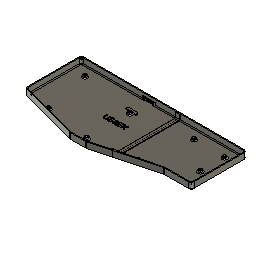
US8EK (Autodesk Fusion 360 design; units mm, degrees)
part number: 2026-03-01-18-28-36-830
Autodesk Fusion 360 part; units mm, degrees
(part 1 of 2)
sketch "Switch plate - imported" plane through (0, 0, 0) normal (0, 0, 1) x (1, 0, 0)
  line L0 (320.63607, 108.23641) -> (-5.90393, 108.23641)
  line L1 (-11.90393, 102.23641) -> (-11.90393, -1.458095)
  line L2 (-7.45498, -7.254149) -> (111.911453, -39.197144)
  line L3 (113.462504, -39.40109) -> (144.22489, -39.40109)
  line L4 (145.76596, -39.199805) -> (270.63368, -6.014874)
  line L5 (272.174751, -5.81359) -> (320.63607, -5.81359)
  line L6 (326.63607, 0.18641) -> (326.63607, 102.23641)
  arc A0 (-5.90393, 108.23641) -> (-11.90393, 102.23641) centre (-5.90393, 102.23641) ccw
  arc A1 (-11.90393, -1.458095) -> (-7.45498, -7.254149) centre (-5.90393, -1.458095) ccw
  arc A2 (111.911453, -39.197144) -> (113.462504, -39.40109) centre (113.462504, -33.40109) ccw
  arc A3 (144.22489, -39.40109) -> (145.76596, -39.199806) centre (144.22489, -33.40109) ccw
  arc A4 (272.174751, -5.81359) -> (270.63368, -6.014874) centre (272.174751, -11.81359) ccw
  arc A5 (320.63607, -5.81359) -> (326.63607, 0.18641) centre (320.63607, 0.18641) ccw
  arc A6 (326.63607, 102.23641) -> (320.63607, 108.23641) centre (320.63607, 102.23641) ccw
  line L7 (-8.820515, -4.494277) -> (4.494277, -8.820515)
  line L8 (4.494277, -8.820515) -> (8.820515, 4.494277)
  line L9 (8.820515, 4.494277) -> (-4.494277, 8.820515)
  line L10 (-4.494277, 8.820515) -> (-8.820515, -4.494277)
  line L11 (-2.949192, 13.575797) -> (10.3656, 9.249559)
  line L12 (10.3656, 9.249559) -> (14.691838, 22.56435)
  line L13 (14.691838, 22.56435) -> (1.377046, 26.890588)
  line L14 (1.377046, 26.890588) -> (-2.949192, 13.575797)
  line L15 (2.922131, 31.645871) -> (16.236923, 27.319633)
  line L16 (16.236923, 27.319633) -> (20.56316, 40.634424)
  line L17 (20.56316, 40.634424) -> (7.248369, 44.960662)
  line L18 (7.248369, 44.960662) -> (2.922131, 31.645871)
  line L19 (8.793454, 49.715945) -> (22.108245, 45.389707)
  line L20 (22.108245, 45.389707) -> (26.434483, 58.704498)
  line L21 (26.434483, 58.704498) -> (13.119692, 63.030736)
  line L22 (13.119692, 63.030736) -> (8.793454, 49.715945)
  line L23 (14.664777, 67.786019) -> (27.979568, 63.459781)
  line L24 (27.979568, 63.459781) -> (32.305806, 76.774572)
  line L25 (32.305806, 76.774572) -> (18.991015, 81.10081)
  line L26 (18.991015, 81.10081) -> (14.664777, 67.786019)
  line L27 (10.426914, -6.742074) -> (23.741705, -11.068312)
  line L28 (23.741705, -11.068312) -> (28.067943, 2.246479)
  line L29 (28.067943, 2.246479) -> (14.753152, 6.572717)
  line L30 (14.753152, 6.572717) -> (10.426914, -6.742074)
  line L31 (16.298237, 11.327999) -> (29.613028, 7.001762)
  line L32 (29.613028, 7.001762) -> (33.939266, 20.316553)
  line L33 (33.939266, 20.316553) -> (20.624475, 24.642791)
  line L34 (20.624475, 24.642791) -> (16.298237, 11.328)
  line L35 (22.16956, 29.398073) -> (35.484351, 25.071836)
  line L36 (35.484351, 25.071836) -> (39.810589, 38.386627)
  line L37 (39.810589, 38.386627) -> (26.495798, 42.712865)
  line L38 (26.495798, 42.712865) -> (22.16956, 29.398073)
  line L39 (28.040883, 47.468147) -> (41.355674, 43.141909)
  line L40 (41.355674, 43.141909) -> (45.681912, 56.456701)
  line L41 (45.681912, 56.456701) -> (32.36712, 60.782939)
  line L42 (32.36712, 60.782939) -> (28.040883, 47.468147)
  line L43 (33.912205, 65.538221) -> (47.226997, 61.211983)
  line L44 (47.226997, 61.211983) -> (51.553235, 74.526774)
  line L45 (51.553235, 74.526774) -> (38.238443, 78.853012)
  line L46 (38.238443, 78.853012) -> (33.912205, 65.538221)
  line L47 (32.617729, 0.068942) -> (45.932521, -4.257296)
  line L48 (45.932521, -4.257296) -> (50.258759, 9.057495)
  line L49 (50.258759, 9.057495) -> (36.943967, 13.383733)
  line L50 (36.943967, 13.383733) -> (32.617729, 0.068941)
  line L51 (38.489052, 18.139015) -> (51.803844, 13.812777)
  line L52 (51.803844, 13.812777) -> (56.130082, 27.127569)
  line L53 (56.130081, 27.127569) -> (42.81529, 31.453807)
  line L54 (42.81529, 31.453807) -> (38.489052, 18.139015)
  line L55 (44.360375, 36.209089) -> (57.675167, 31.882851)
  line L56 (57.675167, 31.882851) -> (62.001404, 45.197643)
  line L57 (62.001404, 45.197643) -> (48.686613, 49.52388)
  line L58 (48.686613, 49.52388) -> (44.360375, 36.209089)
  line L59 (50.231698, 54.279163) -> (63.546489, 49.952925)
  line L60 (63.546489, 49.952925) -> (67.872727, 63.267716)
  line L61 (67.872727, 63.267716) -> (54.557936, 67.593954)
  line L62 (54.557936, 67.593954) -> (50.231698, 54.279163)
  line L63 (56.103021, 72.349237) -> (69.417812, 68.022999)
  line L64 (69.417812, 68.022999) -> (73.74405, 81.33779)
  line L65 (73.74405, 81.33779) -> (60.429259, 85.664028)
  line L66 (60.429259, 85.664028) -> (56.103021, 72.349237)
  line L67 (53.042513, 1.444669) -> (66.357304, -2.881569)
  line L68 (66.357304, -2.881569) -> (70.683542, 10.433223)
  line L69 (70.683542, 10.433223) -> (57.368751, 14.759461)
  line L70 (57.368751, 14.759461) -> (53.042513, 1.444669)
  line L71 (58.913836, 19.514743) -> (72.228627, 15.188505)
  line L72 (72.228627, 15.188505) -> (76.554865, 28.503297)
  line L73 (76.554865, 28.503297) -> (63.240074, 32.829534)
  line L74 (63.240074, 32.829534) -> (58.913836, 19.514743)
  line L75 (64.785158, 37.584817) -> (78.09995, 33.258579)
  line L76 (78.09995, 33.258579) -> (82.426188, 46.57337)
  line L77 (82.426188, 46.57337) -> (69.111396, 50.899608)
  line L78 (69.111396, 50.899608) -> (64.785158, 37.584817)
  line L79 (70.656481, 55.654891) -> (83.971273, 51.328653)
  line L80 (83.971273, 51.328653) -> (88.297511, 64.643444)
  line L81 (88.297511, 64.643444) -> (74.982719, 68.969682)
  line L82 (74.982719, 68.969682) -> (70.656481, 55.654891)
  line L83 (76.527804, 73.724964) -> (89.842596, 69.398727)
  line L84 (89.842596, 69.398727) -> (94.168833, 82.713518)
  line L85 (94.168833, 82.713518) -> (80.854042, 87.039756)
  line L86 (80.854042, 87.039756) -> (76.527804, 73.724964)
  line L87 (68.757877, -11.673704) -> (82.072668, -15.999942)
  line L88 (82.072668, -15.999942) -> (86.398906, -2.685151)
  line L89 (86.398906, -2.685151) -> (73.084115, 1.641087)
  line L90 (73.084115, 1.641087) -> (68.757877, -11.673704)
  line L91 (74.6292, 6.396369) -> (87.943991, 2.070132)
  line L92 (87.943991, 2.070132) -> (92.270229, 15.384923)
  line L93 (92.270229, 15.384923) -> (78.955438, 19.711161)
  line L94 (78.955438, 19.711161) -> (74.6292, 6.396369)
  line L95 (80.500523, 24.466443) -> (93.815314, 20.140205)
  line L96 (93.815314, 20.140205) -> (98.141552, 33.454997)
  line L97 (98.141552, 33.454997) -> (84.826761, 37.781235)
  line L98 (84.826761, 37.781235) -> (80.500523, 24.466443)
  line L99 (86.371846, 42.536517) -> (99.686637, 38.210279)
  line L100 (99.686637, 38.210279) -> (104.012875, 51.52507)
  line L101 (104.012875, 51.525071) -> (90.698084, 55.851308)
  line L102 (90.698084, 55.851308) -> (86.371846, 42.536517)
  line L103 (92.243169, 60.606591) -> (105.55796, 56.280353)
  line L104 (105.55796, 56.280353) -> (109.884198, 69.595144)
  line L105 (109.884198, 69.595144) -> (96.569407, 73.921382)
  line L106 (96.569407, 73.921382) -> (92.243169, 60.606591)
  line L107 (85.650596, -21.168553) -> (98.965387, -25.49479)
  line L108 (98.965387, -25.49479) -> (103.291625, -12.179999)
  line L109 (103.291625, -12.179999) -> (89.976834, -7.853761)
  line L110 (89.976834, -7.853761) -> (85.650596, -21.168553)
  line L111 (91.521919, -3.098479) -> (104.83671, -7.424717)
  line L112 (104.83671, -7.424717) -> (109.162948, 5.890075)
  line L113 (109.162948, 5.890075) -> (95.848157, 10.216313)
  line L114 (95.848157, 10.216313) -> (91.521919, -3.098479)
  line L115 (97.393242, 14.971595) -> (110.708033, 10.645357)
  line L116 (110.708033, 10.645357) -> (115.034271, 23.960148)
  line L117 (115.034271, 23.960148) -> (101.71948, 28.286386)
  line L118 (101.71948, 28.286386) -> (97.393242, 14.971595)
  line L119 (103.264565, 33.041669) -> (116.579356, 28.715431)
  line L120 (116.579356, 28.715431) -> (120.905594, 42.030222)
  line L121 (120.905594, 42.030222) -> (107.590803, 46.35646)
  line L122 (107.590803, 46.35646) -> (103.264565, 33.041669)
  line L123 (109.135888, 51.111743) -> (122.450679, 46.785505)
  line L124 (122.450679, 46.785505) -> (126.776917, 60.100296)
  line L125 (126.776917, 60.100296) -> (113.462125, 64.426534)
  line L126 (113.462125, 64.426534) -> (109.135888, 51.111743)
  line L127 (103.94876, -27.455373) -> (113.316588, -37.8594)
  line L128 (113.316588, -37.8594) -> (123.720616, -28.491572)
  line L129 (123.720616, -28.491572) -> (114.352787, -18.087544)
  line L130 (114.352787, -18.087544) -> (103.94876, -27.455373)
  line L131 (109.050868, -10.797015) -> (122.365659, -15.123253)
  line L132 (122.365659, -15.123253) -> (126.691897, -1.808462)
  line L133 (126.691897, -1.808462) -> (113.377106, 2.517776)
  line L134 (113.377106, 2.517776) -> (109.050868, -10.797015)
  line L135 (-9.37893, 91.71141) -> (4.62107, 91.71141)
  line L136 (4.62107, 91.71141) -> (4.62107, 105.71141)
  line L137 (4.62107, 105.71141) -> (-9.37893, 105.71141)
  line L138 (-9.37893, 105.71141) -> (-9.37893, 91.71141)
  line L139 (13.48107, 91.71141) -> (27.48107, 91.71141)
  line L140 (27.48107, 91.71141) -> (27.48107, 105.71141)
  line L141 (27.48107, 105.71141) -> (13.48107, 105.71141)
  line L142 (13.48107, 105.71141) -> (13.48107, 91.71141)
  line L143 (32.48107, 91.71141) -> (46.48107, 91.71141)
  line L144 (46.48107, 91.71141) -> (46.48107, 105.71141)
  line L145 (46.48107, 105.71141) -> (32.48107, 105.71141)
  line L146 (32.48107, 105.71141) -> (32.48107, 91.71141)
  line L147 (51.48107, 91.71141) -> (65.48107, 91.71141)
  line L148 (65.48107, 91.71141) -> (65.48107, 105.71141)
  line L149 (65.48107, 105.71141) -> (51.48107, 105.71141)
  line L150 (51.48107, 105.71141) -> (51.48107, 91.71141)
  line L151 (70.48107, 91.71141) -> (84.48107, 91.71141)
  line L152 (84.48107, 91.71141) -> (84.48107, 105.71141)
  line L153 (84.48107, 105.71141) -> (70.48107, 105.71141)
  line L154 (70.48107, 105.71141) -> (70.48107, 91.71141)
  line L155 (93.34107, 91.71141) -> (107.34107, 91.71141)
  line L156 (107.34107, 91.71141) -> (107.34107, 105.71141)
  line L157 (107.34107, 105.71141) -> (93.34107, 105.71141)
  line L158 (93.34107, 105.71141) -> (93.34107, 91.71141)
  line L159 (112.34107, 91.71141) -> (126.34107, 91.71141)
  line L160 (126.34107, 91.71141) -> (126.34107, 105.71141)
  line L161 (126.34107, 105.71141) -> (112.34107, 105.71141)
  line L162 (112.34107, 105.71141) -> (112.34107, 91.71141)
  line L163 (131.34107, 91.71141) -> (145.34107, 91.71141)
  line L164 (145.34107, 91.71141) -> (145.34107, 105.71141)
  line L165 (145.34107, 105.71141) -> (131.34107, 105.71141)
  line L166 (131.34107, 105.71141) -> (131.34107, 91.71141)
  line L167 (150.34107, 91.71141) -> (164.34107, 91.71141)
  line L168 (164.34107, 91.71141) -> (164.34107, 105.71141)
  line L169 (164.34107, 105.71141) -> (150.34107, 105.71141)
  line L170 (150.34107, 105.71141) -> (150.34107, 91.71141)
  line L171 (173.20107, 91.71141) -> (187.20107, 91.71141)
  line L172 (187.20107, 91.71141) -> (187.20107, 105.71141)
  line L173 (187.20107, 105.71141) -> (173.20107, 105.71141)
  line L174 (173.20107, 105.71141) -> (173.20107, 91.71141)
  line L175 (192.20107, 91.71141) -> (206.20107, 91.71141)
  line L176 (206.20107, 91.71141) -> (206.20107, 105.71141)
  line L177 (206.20107, 105.71141) -> (192.20107, 105.71141)
  line L178 (192.20107, 105.71141) -> (192.20107, 91.71141)
  line L179 (211.20107, 91.71141) -> (225.20107, 91.71141)
  line L180 (225.20107, 91.71141) -> (225.20107, 105.71141)
  line L181 (225.20107, 105.71141) -> (211.20107, 105.71141)
  line L182 (211.20107, 105.71141) -> (211.20107, 91.71141)
  line L183 (230.20107, 91.71141) -> (244.20107, 91.71141)
  line L184 (244.20107, 91.71141) -> (244.20107, 105.71141)
  line L185 (244.20107, 105.71141) -> (230.20107, 105.71141)
  line L186 (230.20107, 105.71141) -> (230.20107, 91.71141)
  line L187 (272.11107, -3.28859) -> (286.11107, -3.28859)
  line L188 (286.11107, -3.28859) -> (286.11107, 10.71141)
  line L189 (286.11107, 10.71141) -> (272.11107, 10.71141)
  line L190 (272.11107, 10.71141) -> (272.11107, -3.28859)
  line L191 (272.11107, 15.71141) -> (286.11107, 15.71141)
  line L192 (286.11107, 15.71141) -> (286.11107, 29.71141)
  line L193 (286.11107, 29.71141) -> (272.11107, 29.71141)
  line L194 (272.11107, 29.71141) -> (272.11107, 15.71141)
  line L195 (281.63607, 34.71141) -> (295.63607, 34.71141)
  line L196 (295.63607, 34.71141) -> (295.63607, 48.71141)
  line L197 (295.63607, 48.71141) -> (281.63607, 48.71141)
  line L198 (281.63607, 48.71141) -> (281.63607, 34.71141)
  line L199 (272.11107, 53.71141) -> (286.11107, 53.71141)
  line L200 (286.11107, 53.71141) -> (286.11107, 67.71141)
  line L201 (286.11107, 67.71141) -> (272.11107, 67.71141)
  line L202 (272.11107, 67.71141) -> (272.11107, 53.71141)
  line L203 (281.63607, 72.71141) -> (295.63607, 72.71141)
  line L204 (295.63607, 72.71141) -> (295.63607, 86.71141)
  line L205 (295.63607, 86.71141) -> (281.63607, 86.71141)
  line L206 (281.63607, 86.71141) -> (281.63607, 72.71141)
  line L207 (272.11107, 91.71141) -> (286.11107, 91.71141)
  line L208 (286.11107, 91.71141) -> (286.11107, 105.71141)
  line L209 (286.11107, 105.71141) -> (272.11107, 105.71141)
  line L210 (272.11107, 105.71141) -> (272.11107, 91.71141)
  line L211 (291.11107, -3.28859) -> (305.11107, -3.28859)
  line L212 (305.11107, -3.28859) -> (305.11107, 10.71141)
  line L213 (305.11107, 10.71141) -> (291.11107, 10.71141)
  line L214 (291.11107, 10.71141) -> (291.11107, -3.28859)
  line L215 (291.11107, 15.71141) -> (305.11107, 15.71141)
  line L216 (305.11107, 15.71141) -> (305.11107, 29.71141)
  line L217 (305.11107, 29.71141) -> (291.11107, 29.71141)
  line L218 (291.11107, 29.71141) -> (291.11107, 15.71141)
  line L219 (291.11107, 53.71141) -> (305.11107, 53.71141)
  line L220 (305.11107, 53.71141) -> (305.11107, 67.71141)
  line L221 (305.11107, 67.71141) -> (291.11107, 67.71141)
  line L222 (291.11107, 67.71141) -> (291.11107, 53.71141)
  line L223 (291.11107, 91.71141) -> (305.11107, 91.71141)
  line L224 (305.11107, 91.71141) -> (305.11107, 105.71141)
  line L225 (305.11107, 105.71141) -> (291.11107, 105.71141)
  line L226 (291.11107, 105.71141) -> (291.11107, 91.71141)
  line L227 (310.11107, -3.28859) -> (324.11107, -3.28859)
  line L228 (324.11107, -3.28859) -> (324.11107, 10.71141)
  line L229 (324.11107, 10.71141) -> (310.11107, 10.71141)
  line L230 (310.11107, 10.71141) -> (310.11107, -3.28859)
  line L231 (310.11107, 15.71141) -> (324.11107, 15.71141)
  line L232 (324.11107, 15.71141) -> (324.11107, 29.71141)
  line L233 (324.11107, 29.71141) -> (310.11107, 29.71141)
  line L234 (310.11107, 29.71141) -> (310.11107, 15.71141)
  line L235 (310.11107, 34.71141) -> (324.11107, 34.71141)
  line L236 (324.11107, 34.71141) -> (324.11107, 48.71141)
  line L237 (324.11107, 48.71141) -> (310.11107, 48.71141)
  line L238 (310.11107, 48.71141) -> (310.11107, 34.71141)
  line L239 (310.11107, 53.71141) -> (324.11107, 53.71141)
  line L240 (324.11107, 53.71141) -> (324.11107, 67.71141)
  line L241 (324.11107, 67.71141) -> (310.11107, 67.71141)
  line L242 (310.11107, 67.71141) -> (310.11107, 53.71141)
  line L243 (310.11107, 72.71141) -> (324.11107, 72.71141)
  line L244 (324.11107, 72.71141) -> (324.11107, 86.71141)
  line L245 (324.11107, 86.71141) -> (310.11107, 86.71141)
  line L246 (310.11107, 86.71141) -> (310.11107, 72.71141)
  line L247 (310.11107, 91.71141) -> (324.11107, 91.71141)
  line L248 (324.11107, 91.71141) -> (324.11107, 105.71141)
  line L249 (324.11107, 105.71141) -> (310.11107, 105.71141)
  line L250 (310.11107, 105.71141) -> (310.11107, 91.71141)
  line L251 (-9.37893, 53.61141) -> (4.62107, 53.61141)
  line L252 (4.62107, 53.61141) -> (4.62107, 67.61141)
  line L253 (4.62107, 67.61141) -> (-9.37893, 67.61141)
  line L254 (-9.37893, 67.61141) -> (-9.37893, 53.61141)
  line L255 (-9.37893, 72.61141) -> (4.62107, 72.61141)
  line L256 (4.62107, 72.61141) -> (4.62107, 86.61141)
  line L257 (4.62107, 86.61141) -> (-9.37893, 86.61141)
  line L258 (-9.37893, 86.61141) -> (-9.37893, 72.61141)
  line L259 (255.305035, 48.586497) -> (268.619826, 52.912735)
  line L260 (268.619826, 52.912735) -> (264.293588, 66.227526)
  line L261 (264.293588, 66.227526) -> (250.978797, 61.901288)
  line L262 (250.978797, 61.901288) -> (255.305035, 48.586497)
  line L263 (249.433712, 66.656571) -> (262.748503, 70.982809)
  line L264 (262.748503, 70.982809) -> (258.422265, 84.2976)
  line L265 (258.422265, 84.2976) -> (245.107474, 79.971362)
  line L266 (245.107474, 79.971362) -> (249.433712, 66.656571)
  line L267 (253.06107, 91.71141) -> (267.06107, 91.71141)
  line L268 (267.06107, 91.71141) -> (267.06107, 105.71141)
  line L269 (267.06107, 105.71141) -> (253.06107, 105.71141)
  line L270 (253.06107, 105.71141) -> (253.06107, 91.71141)
  line L271 (121.86607, 7.89141) -> (135.86607, 7.89141)
  line L272 (135.86607, 7.89141) -> (135.86607, 21.89141)
  line L273 (135.86607, 21.89141) -> (121.86607, 21.89141)
  line L274 (121.86607, 21.89141) -> (121.86607, 7.89141)
  line L275 (112.34107, 72.66141) -> (126.34107, 72.66141)
  line L276 (126.34107, 72.66141) -> (126.34107, 86.66141)
  line L277 (126.34107, 86.66141) -> (112.34107, 86.66141)
  line L278 (112.34107, 86.66141) -> (112.34107, 72.66141)
  line L279 (131.34107, 72.66141) -> (145.34107, 72.66141)
  line L280 (145.34107, 72.66141) -> (145.34107, 86.66141)
  line L281 (145.34107, 86.66141) -> (131.34107, 86.66141)
  line L282 (131.34107, 86.66141) -> (131.34107, 72.66141)
  line L283 (253.933236, -8.820515) -> (267.248028, -4.494277)
  line L284 (267.248028, -4.494277) -> (262.92179, 8.820515)
  line L285 (262.92179, 8.820515) -> (249.606998, 4.494277)
  line L286 (249.606998, 4.494277) -> (253.933236, -8.820515)
  line L287 (248.061913, 9.249559) -> (261.376705, 13.575797)
  line L288 (261.376705, 13.575797) -> (257.050467, 26.890588)
  line L289 (257.050467, 26.890588) -> (243.735676, 22.56435)
  line L290 (243.735676, 22.56435) -> (248.061913, 9.249559)
  line L291 (242.19059, 27.319633) -> (255.505382, 31.645871)
  line L292 (255.505382, 31.645871) -> (251.179144, 44.960662)
  line L293 (251.179144, 44.960662) -> (237.864353, 40.634424)
  line L294 (237.864353, 40.634424) -> (242.19059, 27.319633)
  line L295 (236.319268, 45.389707) -> (249.634059, 49.715945)
  line L296 (249.634059, 49.715945) -> (245.307821, 63.030736)
  line L297 (245.307821, 63.030736) -> (231.99303, 58.704498)
  line L298 (231.99303, 58.704498) -> (236.319268, 45.389707)
  line L299 (230.447945, 63.459781) -> (243.762736, 67.786019)
  line L300 (243.762736, 67.786019) -> (239.436498, 81.10081)
  line L301 (239.436498, 81.10081) -> (226.121707, 76.774572)
  line L302 (226.121707, 76.774572) -> (230.447945, 63.459781)
  line L303 (234.685808, -11.068312) -> (248.000599, -6.742074)
  line L304 (248.000599, -6.742074) -> (243.674361, 6.572717)
  line L305 (243.674361, 6.572717) -> (230.35957, 2.246479)
  line L306 (230.35957, 2.246479) -> (234.685808, -11.068312)
  line L307 (228.814485, 7.001762) -> (242.129276, 11.327999)
  line L308 (242.129276, 11.327999) -> (237.803038, 24.642791)
  line L309 (237.803038, 24.642791) -> (224.488247, 20.316553)
  line L310 (224.488247, 20.316553) -> (228.814485, 7.001762)
  line L311 (222.943162, 25.071836) -> (236.257953, 29.398073)
  line L312 (236.257953, 29.398073) -> (231.931715, 42.712865)
  line L313 (231.931715, 42.712865) -> (218.616924, 38.386627)
  line L314 (218.616924, 38.386627) -> (222.943162, 25.071836)
  line L315 (217.071839, 43.141909) -> (230.38663, 47.468147)
  line L316 (230.38663, 47.468147) -> (226.060392, 60.782939)
  line L317 (226.060392, 60.782939) -> (212.745601, 56.456701)
  line L318 (212.745601, 56.456701) -> (217.071839, 43.141909)
  line L319 (211.200516, 61.211983) -> (224.515308, 65.538221)
  line L320 (224.515308, 65.538221) -> (220.18907, 78.853012)
  line L321 (220.18907, 78.853012) -> (206.874278, 74.526774)
  line L322 (206.874278, 74.526774) -> (211.200516, 61.211983)
  line L323 (212.494992, -4.257296) -> (225.809784, 0.068942)
  line L324 (225.809784, 0.068941) -> (221.483546, 13.383733)
  line L325 (221.483546, 13.383733) -> (208.168754, 9.057495)
  line L326 (208.168754, 9.057495) -> (212.494992, -4.257296)
  line L327 (206.623669, 13.812777) -> (219.938461, 18.139015)
  line L328 (219.938461, 18.139015) -> (215.612223, 31.453807)
  line L329 (215.612223, 31.453807) -> (202.297432, 27.127569)
  line L330 (202.297432, 27.127569) -> (206.623669, 13.812777)
  line L331 (200.752347, 31.882851) -> (214.067138, 36.209089)
  line L332 (214.067138, 36.209089) -> (209.7409, 49.52388)
  line L333 (209.7409, 49.52388) -> (196.426109, 45.197643)
  line L334 (196.426109, 45.197643) -> (200.752347, 31.882851)
  line L335 (194.881024, 49.952925) -> (208.195815, 54.279163)
  line L336 (208.195815, 54.279163) -> (203.869577, 67.593954)
  line L337 (203.869577, 67.593954) -> (190.554786, 63.267716)
  line L338 (190.554786, 63.267716) -> (194.881024, 49.952925)
  line L339 (189.009701, 68.022999) -> (202.324492, 72.349237)
  line L340 (202.324492, 72.349237) -> (197.998254, 85.664028)
  line L341 (197.998254, 85.664028) -> (184.683463, 81.33779)
  line L342 (184.683463, 81.33779) -> (189.009701, 68.022999)
  line L343 (192.070209, -2.881569) -> (205.385, 1.444669)
  line L344 (205.385, 1.444669) -> (201.058762, 14.759461)
  line L345 (201.058762, 14.759461) -> (187.743971, 10.433223)
  line L346 (187.743971, 10.433223) -> (192.070209, -2.881569)
  line L347 (186.198886, 15.188505) -> (199.513677, 19.514743)
  line L348 (199.513677, 19.514743) -> (195.187439, 32.829534)
  line L349 (195.18744, 32.829534) -> (181.872648, 28.503297)
  line L350 (181.872648, 28.503297) -> (186.198886, 15.188505)
  line L351 (180.327563, 33.258579) -> (193.642355, 37.584817)
  line L352 (193.642354, 37.584817) -> (189.316117, 50.899608)
  line L353 (189.316117, 50.899608) -> (176.001325, 46.57337)
  line L354 (176.001325, 46.57337) -> (180.327563, 33.258579)
  line L355 (174.45624, 51.328653) -> (187.771032, 55.654891)
  line L356 (187.771032, 55.654891) -> (183.444794, 68.969682)
  line L357 (183.444794, 68.969682) -> (170.130002, 64.643444)
  line L358 (170.130002, 64.643444) -> (174.45624, 51.328653)
  line L359 (168.584917, 69.398727) -> (181.899709, 73.724964)
  line L360 (181.899709, 73.724964) -> (177.573471, 87.039756)
  line L361 (177.573471, 87.039756) -> (164.258679, 82.713518)
  line L362 (164.258679, 82.713518) -> (168.584917, 69.398727)
  line L363 (176.354845, -15.999942) -> (189.669636, -11.673704)
  line L364 (189.669636, -11.673704) -> (185.343398, 1.641087)
  line L365 (185.343398, 1.641087) -> (172.028607, -2.685151)
  line L366 (172.028607, -2.685151) -> (176.354845, -15.999942)
  line L367 (170.483522, 2.070132) -> (183.798313, 6.39637)
  line L368 (183.798313, 6.396369) -> (179.472075, 19.711161)
  line L369 (179.472075, 19.711161) -> (166.157284, 15.384923)
  line L370 (166.157284, 15.384923) -> (170.483522, 2.070132)
  line L371 (164.612199, 20.140205) -> (177.92699, 24.466443)
  line L372 (177.92699, 24.466443) -> (173.600752, 37.781235)
  line L373 (173.600752, 37.781235) -> (160.285961, 33.454997)
  line L374 (160.285961, 33.454997) -> (164.612199, 20.140205)
  line L375 (158.740876, 38.210279) -> (172.055667, 42.536517)
  line L376 (172.055667, 42.536517) -> (167.729429, 55.851308)
  line L377 (167.729429, 55.851308) -> (154.414638, 51.525071)
  line L378 (154.414638, 51.525071) -> (158.740876, 38.210279)
  line L379 (152.869553, 56.280353) -> (166.184344, 60.606591)
  line L380 (166.184344, 60.606591) -> (161.858107, 73.921382)
  line L381 (161.858107, 73.921382) -> (148.543315, 69.595144)
  line L382 (148.543315, 69.595144) -> (152.869553, 56.280353)
  line L383 (159.462126, -25.49479) -> (172.776917, -21.168552)
  line L384 (172.776917, -21.168553) -> (168.450679, -7.853761)
  line L385 (168.450679, -7.853761) -> (155.135888, -12.179999)
  line L386 (155.135888, -12.179999) -> (159.462126, -25.49479)
  line L387 (153.590803, -7.424717) -> (166.905594, -3.098479)
  line L388 (166.905594, -3.098479) -> (162.579356, 10.216313)
  line L389 (162.579356, 10.216313) -> (149.264565, 5.890075)
  line L390 (149.264565, 5.890075) -> (153.590803, -7.424717)
  line L391 (147.71948, 10.645357) -> (161.034271, 14.971595)
  line L392 (161.034271, 14.971595) -> (156.708033, 28.286386)
  line L393 (156.708033, 28.286386) -> (143.393242, 23.960148)
  line L394 (143.393242, 23.960148) -> (147.71948, 10.645357)
  line L395 (141.848157, 28.715431) -> (155.162948, 33.041669)
  line L396 (155.162948, 33.041669) -> (150.83671, 46.35646)
  line L397 (150.83671, 46.35646) -> (137.521919, 42.030222)
  line L398 (137.521919, 42.030222) -> (141.848157, 28.715431)
  line L399 (135.976834, 46.785505) -> (149.291625, 51.111743)
  line L400 (149.291625, 51.111743) -> (144.965387, 64.426534)
  line L401 (144.965387, 64.426534) -> (131.650596, 60.100296)
  line L402 (131.650596, 60.100296) -> (135.976834, 46.785505)
  line L403 (145.110925, -37.8594) -> (154.478753, -27.455373)
  line L404 (154.478753, -27.455373) -> (144.074726, -18.087544)
  line L405 (144.074726, -18.087544) -> (134.706897, -28.491572)
  line L406 (134.706897, -28.491572) -> (145.110925, -37.8594)
  line L407 (136.061853, -15.123253) -> (149.376645, -10.797015)
  line L408 (149.376645, -10.797015) -> (145.050407, 2.517776)
  line L409 (145.050407, 2.517776) -> (131.735616, -1.808462)
  line L410 (131.735616, -1.808462) -> (136.061853, -15.123253)
  circle A7 centre (17.958543, 86.094258) radius 1.2
  circle A8 centre (37.317502, -8.11912) radius 1.2
  circle A9 centre (128.86607, -21.30359) radius 1.2
  circle A10 centre (128.86607, 66.32641) radius 1.2
  circle A11 centre (240.468971, 86.094258) radius 1.2
  circle A12 centre (221.110011, -8.11912) radius 1.2
  circle A13 centre (303.77607, 85.42641) radius 1.2
  circle A14 centre (303.77607, 35.99641) radius 1.2
  line L411 (-9.90393, 102.23641) -> (-9.90393, -1.458095)
  arc A15 (-9.90393, -1.458095) -> (-6.937964, -5.322131) centre (-5.90393, -1.458095) ccw
  line L412 (-6.937964, -5.322131) -> (112.42847, -37.265126)
  arc A16 (112.42847, -37.265126) -> (113.462504, -37.40109) centre (113.462504, -33.40109) ccw
  line L413 (113.462504, -37.40109) -> (144.22489, -37.40109)
  arc A17 (144.22489, -37.40109) -> (145.25227, -37.2669) centre (144.22489, -33.40109) ccw
  line L414 (145.25227, -37.2669) -> (270.11999, -4.081969)
  arc A18 (272.174751, -3.81359) -> (270.11999, -4.081969) centre (272.174751, -11.81359) ccw
  line L415 (272.174751, -3.81359) -> (320.63607, -3.81359)
  arc A19 (320.63607, -3.81359) -> (324.63607, 0.18641) centre (320.63607, 0.18641) ccw
  line L416 (324.63607, 0.18641) -> (324.63607, 102.23641)
  arc A20 (324.63607, 102.23641) -> (320.63607, 106.23641) centre (320.63607, 102.23641) ccw
  line L417 (320.63607, 106.23641) -> (-5.90393, 106.23641)
  arc A21 (-5.90393, 106.23641) -> (-9.90393, 102.23641) centre (-5.90393, 102.23641) ccw
  dimension "wall_thickness" = -2
sketch "Case - top down" plane through (0, 0, 0) normal (0, 0, 1) x (1, 0, 0)
  line L0 (-9.90393, 102.23641) -> (-9.90393, -1.458095)
  line L1 (-11.90393, 102.23641) -> (-11.90393, -1.458095)
  arc A0 (-11.90393, -1.458095) -> (-7.45498, -7.254149) centre (-5.90393, -1.458095) ccw
  arc A1 (-9.90393, -1.458095) -> (-6.937964, -5.322131) centre (-5.90393, -1.458095) ccw
  line L2 (-6.937964, -5.322131) -> (112.42847, -37.265126)
  line L3 (-7.45498, -7.254149) -> (111.911453, -39.197144)
  arc A2 (-5.90393, 106.23641) -> (-9.90393, 102.23641) centre (-5.90393, 102.23641) ccw
  arc A3 (-5.90393, 108.23641) -> (-11.90393, 102.23641) centre (-5.90393, 102.23641) ccw
  line L4 (320.63607, 106.23641) -> (-5.90393, 106.23641)
  line L5 (320.63607, 108.23641) -> (-5.90393, 108.23641)
  line L6 (113.462504, -37.40109) -> (144.22489, -37.40109)
  line L7 (113.462504, -39.40109) -> (144.22489, -39.40109)
  arc A4 (111.911453, -39.197144) -> (113.462504, -39.40109) centre (113.462504, -33.40109) ccw
  arc A5 (112.42847, -37.265126) -> (113.462504, -37.40109) centre (113.462504, -33.40109) ccw
  arc A6 (144.22489, -39.40109) -> (145.76596, -39.199806) centre (144.22489, -33.40109) ccw
  line L8 (145.76596, -39.199805) -> (270.63368, -6.014874)
  line L9 (145.25227, -37.2669) -> (270.11999, -4.081969)
  arc A7 (144.22489, -37.40109) -> (145.25227, -37.2669) centre (144.22489, -33.40109) ccw
  arc A8 (272.174751, -3.81359) -> (270.11999, -4.081969) centre (272.174751, -11.81359) ccw
  arc A9 (272.174751, -5.81359) -> (270.63368, -6.014874) centre (272.174751, -11.81359) ccw
  line L10 (272.174751, -5.81359) -> (320.63607, -5.81359)
  line L11 (272.174751, -3.81359) -> (320.63607, -3.81359)
  arc A10 (320.63607, -5.81359) -> (326.63607, 0.18641) centre (320.63607, 0.18641) ccw
  arc A11 (320.63607, -3.81359) -> (324.63607, 0.18641) centre (320.63607, 0.18641) ccw
  line L12 (324.63607, 0.18641) -> (324.63607, 102.23641)
  line L13 (326.63607, 0.18641) -> (326.63607, 102.23641)
  arc A12 (326.63607, 102.23641) -> (320.63607, 108.23641) centre (320.63607, 102.23641) ccw
  arc A13 (324.63607, 102.23641) -> (320.63607, 106.23641) centre (320.63607, 102.23641) ccw
sketch "Case - side" plane through (0, 0, 0) normal (1, 0, 0) x (0, 1, 0)
  line L0 (102.23641, 0) -> (-1.458095, 0) construction
  line L1 (-1.458095, 0) -> (-1.458095, 12)
  line L2 (-1.458095, 0) -> (-1.458095, -1.4)
  point P0 (-1.458095, 4)
  dimension "d2" = 12
  dimension "d3" = 1.4
  dimension "d28" = 4
  constraint perpendicular L0 L1
  constraint perpendicular L0 L2
extrude "Extrude1" add sketch "Case - top down" against normal up to surface (1.4 mm away) contours L0 A1 L2 A2 L4 L6 A5 L9 A7 A8 L11 A11 L12 A13 | L1 A0 L3 A3 L5 L7 A4 A6 L8 A9 L10 A10 L13 A12 picked at (153.328137, 58.401973) picked at (102.942737, 107.569743) makes body 1
extrude "Extrude2" add sketch "Case - top down" along normal up to surface (12 mm away) contours L1 A0 L3 A3 L5 L7 A4 A6 L8 A9 L10 A10 L13 A12 picked at (102.942737, 107.569743) bodies 1
sketch "Overlapping switches - top down" plane through (0, 0, 0) normal (0, 0, 1) x (-1, 0, 0)
  line L0 (6.937964, 5.322131) -> (-112.42847, 37.265126) construction
  arc A0 (-112.42847, 37.265126) -> (-113.462504, 37.40109) centre (-113.462504, 33.40109) ccw construction
  line L1 (-113.462504, 37.40109) -> (-144.22489, 37.40109) construction
  arc A1 (-144.22489, 37.40109) -> (-145.25227, 37.2669) centre (-144.22489, 33.40109) ccw construction
  line L2 (-145.25227, 37.2669) -> (-270.11999, 4.081969) construction
  arc A2 (-272.174751, 3.81359) -> (-270.11999, 4.081969) centre (-272.174751, 11.81359) ccw construction
  line L3 (-272.174751, 3.81359) -> (-320.63607, 3.81359) construction
  arc A3 (-320.63607, 3.81359) -> (-324.63607, -0.18641) centre (-320.63607, -0.18641) ccw construction
  line L4 (-324.63607, -0.18641) -> (-324.63607, -102.23641) construction
  arc A4 (-324.63607, -102.23641) -> (-320.63607, -106.23641) centre (-320.63607, -102.23641) ccw construction
  line L5 (-320.63607, -106.23641) -> (5.90393, -106.23641) construction
  arc A5 (5.90393, -106.23641) -> (9.90393, -102.23641) centre (5.90393, -102.23641) ccw construction
  line L6 (9.90393, -102.23641) -> (9.90393, 1.458095) construction
  arc A6 (9.90393, 1.458095) -> (6.937964, 5.322131) centre (5.90393, 1.458095) ccw construction
  line L7 (4.494277, -8.820515) -> (8.820515, 4.494277) construction
  line L8 (-8.820515, -4.494277) -> (4.494277, -8.820515) construction
  line L9 (-4.494277, 8.820515) -> (-8.820515, -4.494277) construction
  line L10 (8.820515, 4.494277) -> (-4.494277, 8.820515) construction
  line L11 (-4.62107, -105.71141) -> (9.37893, -105.71141) construction
  line L12 (9.37893, -105.71141) -> (9.37893, -91.71141) construction
  line L13 (9.37893, -91.71141) -> (-4.62107, -91.71141) construction
  line L14 (-4.62107, -91.71141) -> (-4.62107, -105.71141) construction
  line L15 (-324.11107, -105.71141) -> (-310.11107, -105.71141) construction
  line L16 (-324.11107, -91.71141) -> (-324.11107, -105.71141) construction
  line L17 (-310.11107, -91.71141) -> (-324.11107, -91.71141) construction
  line L18 (-310.11107, -105.71141) -> (-310.11107, -91.71141) construction
  line L19 (-310.11107, 3.28859) -> (-324.11107, 3.28859) construction
  line L20 (-324.11107, 3.28859) -> (-324.11107, -10.71141) construction
  line L21 (-324.11107, -10.71141) -> (-310.11107, -10.71141) construction
  line L22 (-310.11107, -10.71141) -> (-310.11107, 3.28859) construction
  line L23 (-267.248028, 4.494277) -> (-262.92179, -8.820515) construction
  line L24 (-249.606998, -4.494277) -> (-253.933236, 8.820515) construction
  line L25 (-262.92179, -8.820515) -> (-249.606998, -4.494277) construction
  line L26 (-253.933236, 8.820515) -> (-267.248028, 4.494277) construction
  line L27 (-103.94876, 27.455373) -> (-113.316588, 37.8594) construction
  line L28 (-113.316588, 37.8594) -> (-123.720616, 28.491572) construction
  line L29 (-123.720616, 28.491572) -> (-114.352787, 18.087544) construction
  line L30 (-114.352787, 18.087544) -> (-103.94876, 27.455373) construction
  line L31 (-134.706897, 28.491572) -> (-145.110925, 37.8594) construction
  line L32 (-144.074726, 18.087544) -> (-134.706897, 28.491572) construction
  line L33 (-154.478753, 27.455373) -> (-144.074726, 18.087544) construction
  line L34 (-145.110925, 37.8594) -> (-154.478753, 27.455373) construction
  line L35 (-4.92107, -91.41141) -> (-4.92107, -106.01141)
  line L36 (-4.92107, -106.01141) -> (9.67893, -106.01141)
  line L37 (9.67893, -106.01141) -> (9.67893, -91.41141)
  line L38 (9.67893, -91.41141) -> (-4.92107, -91.41141)
  line L39 (-9.198537, -4.686889) -> (4.686889, -9.198537)
  line L40 (4.686889, -9.198537) -> (9.198537, 4.686889)
  line L41 (9.198537, 4.686889) -> (-4.686889, 9.198537)
  line L42 (-4.686889, 9.198537) -> (-9.198537, -4.686889)
  line L43 (-103.525077, 27.433169) -> (-112.710723, 37.634862)
  line L44 (-112.710723, 37.634862) -> (-113.294384, 38.283083)
  line L45 (-113.294384, 38.283083) -> (-124.144299, 28.513776)
  line L46 (-124.144299, 28.513776) -> (-114.374992, 17.663862)
  line L47 (-114.374992, 17.663862) -> (-103.525077, 27.433169)
  line L48 (-134.283214, 28.513776) -> (-144.47845, 37.693608)
  line L49 (-144.47845, 37.693608) -> (-145.133129, 38.283083)
  line L50 (-145.133129, 38.283083) -> (-154.902436, 27.433169)
  line L51 (-154.902436, 27.433169) -> (-144.052521, 17.663862)
  line L52 (-144.052521, 17.663862) -> (-134.283214, 28.513776)
  line L53 (-253.740624, 9.198537) -> (-267.62605, 4.686889)
  line L54 (-267.62605, 4.686889) -> (-263.114402, -9.198537)
  line L55 (-263.114402, -9.198537) -> (-249.228976, -4.686889)
  line L56 (-249.228976, -4.686889) -> (-253.740624, 9.198537)
  line L57 (-309.81107, 3.58859) -> (-322.695044, 3.58859)
  line L58 (-322.695044, 3.58859) -> (-324.41107, 3.58859)
  line L59 (-324.41107, 3.58859) -> (-324.41107, 1.872564)
  line L60 (-324.41107, 1.872564) -> (-324.41107, -11.01141)
  line L61 (-324.41107, -11.01141) -> (-309.81107, -11.01141)
  line L62 (-309.81107, -11.01141) -> (-309.81107, 3.58859)
  line L63 (-324.41107, -91.41141) -> (-324.41107, -104.295384)
  line L64 (-324.41107, -104.295384) -> (-324.41107, -106.01141)
  line L65 (-324.41107, -106.01141) -> (-322.695044, -106.01141)
  line L66 (-322.695044, -106.01141) -> (-309.81107, -106.01141)
  line L67 (-309.81107, -106.01141) -> (-309.81107, -91.41141)
  line L68 (-309.81107, -91.41141) -> (-324.41107, -91.41141)
  dimension "d30" = 0.3
  dimension "d31" = 0.3
  dimension "d34" = 0.3
  dimension "d35" = 0.3
  dimension "d36" = 0.3
  dimension "d37" = 0.3
  dimension "d38" = 0.3
extrude "Extrude4" cut sketch "Overlapping switches - top down" against normal blind 4 from surface at 12 contours L35 L36 L37 L38 | L39 L40 L41 L42 | L43 L44 L45 L46 L47 | L48 L49 L50 L51 L52 | L53 L54 L55 L56 | L57 L58 L59 L60 L61 L62 | L63 L64 L65 L66 L67 L68 picked at (-0.054403, -101.144743) picked at (-1.562296, 3.066179) picked at (-117.076671, 27.9375) picked at (-147.811136, 27.596879) picked at (-261.493692, 1.562296) picked at (-314.105728, -1.278077) picked at (-319.544403, -95.706068) bodies 1
sketch "Heat sinks - top down" plane through (0, 0, 0) normal (0, 0, 1) x (-1, 0, 0)
  line L0 (6.937964, 5.322131) -> (-112.42847, 37.265126)
  line L1 (-113.462504, 37.40109) -> (-144.22489, 37.40109)
  line L2 (-145.25227, 37.2669) -> (-270.11999, 4.081969)
  arc A0 (-272.174751, 3.81359) -> (-270.11999, 4.081969) centre (-272.174751, 11.81359) ccw
  line L3 (-272.174751, 3.81359) -> (-320.63607, 3.81359)
  arc A1 (-320.63607, 3.81359) -> (-324.63607, -0.18641) centre (-320.63607, -0.18641) ccw
  line L4 (-324.63607, -0.18641) -> (-324.63607, -102.23641)
  arc A2 (-324.63607, -102.23641) -> (-320.63607, -106.23641) centre (-320.63607, -102.23641) ccw
  line L5 (-320.63607, -106.23641) -> (5.90393, -106.23641)
  arc A3 (5.90393, -106.23641) -> (9.90393, -102.23641) centre (5.90393, -102.23641) ccw
  line L6 (9.90393, -102.23641) -> (9.90393, 1.458095)
  arc A4 (9.90393, 1.458095) -> (6.937964, 5.322131) centre (5.90393, 1.458095) ccw
  circle A5 centre (-17.958543, -86.094258) radius 1.75
  circle A6 centre (-37.317502, 8.11912) radius 1.75
  circle A7 centre (-128.86607, -66.32641) radius 1.75
  circle A8 centre (-240.468971, -86.094258) radius 1.75
  circle A9 centre (-221.110011, 8.11912) radius 1.75
  circle A10 centre (-303.77607, -35.99641) radius 1.75
  circle A11 centre (-303.77607, -85.42641) radius 1.75
  circle A12 centre (-128.86607, 21.30359) radius 1.75
  circle A13 centre (-17.958543, -86.094258) radius 3.55
  circle A14 centre (-37.317502, 8.11912) radius 3.55
  circle A15 centre (-128.86607, -66.32641) radius 3.55
  circle A16 centre (-128.86607, 21.30359) radius 3.55
  circle A17 centre (-221.110011, 8.11912) radius 3.55
  circle A18 centre (-303.77607, -35.99641) radius 3.55
  circle A19 centre (-303.77607, -85.42641) radius 3.55
  circle A20 centre (-240.468971, -86.094258) radius 3.55
  arc A21 (-112.42847, 37.265126) -> (-113.462504, 37.40109) centre (-113.462504, 33.40109) ccw
  arc A22 (-144.22489, 37.40109) -> (-145.25227, 37.2669) centre (-144.22489, 33.40109) ccw
  point P0 (-17.958543, -86.094258)
  point P1 (-37.317502, 8.11912)
  point P2 (-128.86607, 21.30359)
  point P3 (-128.86607, -66.32641)
  point P4 (-221.110011, 8.11912)
  point P5 (-303.77607, -35.99641)
  point P6 (-303.77607, -85.42641)
  point P7 (-240.468971, -86.094258)
  dimension "d10" = 3.5
  dimension "d11" = 3.5
  dimension "d12" = 3.5
  dimension "d13" = 3.5
  dimension "d14" = 3.5
  dimension "d15" = 3.5
  dimension "d16" = 3.5
  dimension "d17" = 3.5
  dimension "d18" = 1.8
  dimension "d21" = 1.8
  dimension "d22" = 1.8
  dimension "d23" = 1.8
  dimension "d24" = 1.8
  dimension "d25" = 1.8
  dimension "d26" = 1.8
  dimension "d27" = 1.8
  constraint concentric A6 A14
  constraint concentric A11 A19
  measures "d10" diameter of A5
  measures "d11" diameter of A10
  measures "d12" diameter of A11
  measures "d13" diameter of A12
  measures "d14" diameter of A7
  measures "d15" diameter of A6
  measures "d16" diameter of A8
  measures "d17" diameter of A9
  measures "d18" distance of A5 A13
  measures "d21" distance of A6 A14
  measures "d22" distance of A7 A15
  measures "d23" distance of A12 A16
  measures "d24" distance of A9 A17
  measures "d25" distance of A8 A20
  measures "d26" distance of A11 A19
  measures "d27" distance of A10 A18
extrude "Extrude3" add sketch "Heat sinks - top down" along normal up to surface (4 mm away) contours A13 | A14 | A15 | A16 | A17 | A18 | A19 | A20 picked at (-15.028275, -86.357566) picked at (-34.387235, 7.855812) picked at (-127.957318, -63.528202) picked at (-127.957318, 18.505382) picked at (-218.173227, 7.942754) picked at (-302.867318, -33.198202) picked at (-302.867318, -88.224618) picked at (-243.405754, -86.270625) bodies 1
sketch "UCB-C cutout - profile" plane through (0, 106.23641, 0) normal (0, -1, 0) x (1, 0, 0)
  line L0 (320.63607, 12) -> (-5.90393, 12) construction
  line L1 (-5.90393, 12) -> (-5.90393, 0) construction
  line L2 (-5.90393, 0) -> (320.63607, 0) construction
  line L3 (320.63607, 0) -> (320.63607, 12) construction
  line L4 (128.86607, 0) -> (128.86607, 12) construction
  line L5 (123.77607, 5.25) -> (133.95607, 5.25)
  line L6 (133.95607, 5.25) -> (133.95607, 0.6)
  line L7 (133.95607, 0.6) -> (123.77607, 0.6)
  line L8 (123.77607, 0.6) -> (123.77607, 5.25)
  point P0 (128.86607, 0)
  point P1 (128.86607, 0.6)
  dimension "d73" = 0.6
  dimension "d74" = 4.65
  dimension "d75" = 10.18
  constraint perpendicular L2 L4
  constraint parallel L5 L7
  constraint parallel L6 L8
  constraint parallel L2 L7
  constraint perpendicular L6 L7
  measures "d73" distance of L2 L7
extrude "Extrude9" cut sketch "UCB-C cutout - profile" against normal up to surface (2 mm away) contours L5 L6 L7 L8 picked at (130.562737, 3.7) bodies 1
sketch "UCB-C cutout - fillet removal - profile" plane through (0, 0, 0) normal (0, 0, 1) x (-1, 0, 0)
  circle A0 centre (-128.86607, 21.30359) radius 3.55
  circle A1 centre (-221.110011, 8.11912) radius 3.55
  circle A2 centre (-128.86607, -66.32641) radius 3.55
  circle A3 centre (-240.468971, -86.094258) radius 3.55
  line L0 (6.937964, 5.322131) -> (-112.42847, 37.265126)
  arc A4 (-112.42847, 37.265126) -> (-113.462504, 37.40109) centre (-113.462504, 33.40109) ccw
  line L1 (-113.462504, 37.40109) -> (-144.22489, 37.40109)
  arc A5 (-144.22489, 37.40109) -> (-145.25227, 37.2669) centre (-144.22489, 33.40109) ccw
  line L2 (-145.25227, 37.2669) -> (-270.11999, 4.081969)
  arc A6 (-272.174751, 3.81359) -> (-270.11999, 4.081969) centre (-272.174751, 11.81359) ccw
  line L3 (-272.174751, 3.81359) -> (-320.63607, 3.81359)
  arc A7 (-320.63607, 3.81359) -> (-324.63607, -0.18641) centre (-320.63607, -0.18641) ccw
  line L4 (-324.63607, -0.18641) -> (-324.63607, -102.23641)
  arc A8 (-324.63607, -102.23641) -> (-320.63607, -106.23641) centre (-320.63607, -102.23641) ccw
  line L5 (-320.63607, -106.23641) -> (5.90393, -106.23641)
  arc A9 (5.90393, -106.23641) -> (9.90393, -102.23641) centre (5.90393, -102.23641) ccw
  line L6 (9.90393, -102.23641) -> (9.90393, 1.458095)
  arc A10 (9.90393, 1.458095) -> (6.937964, 5.322131) centre (5.90393, 1.458095) ccw
  circle A11 centre (-37.317502, 8.11912) radius 3.55
  circle A12 centre (-303.77607, -85.42641) radius 3.55
  circle A13 centre (-17.958543, -86.094258) radius 3.55
  circle A14 centre (-303.77607, -35.99641) radius 3.55
  line L7 (-133.95607, -106.23641) -> (-123.77607, -106.23641)
  line L8 (-320.63607, -106.23641) -> (5.90393, -106.23641)
  line L9 (-119.86607, -106.23641) -> (-119.86607, -73.23641) construction
  line L10 (-119.86607, -73.23641) -> (-128.86607, -73.23641) construction
  line L11 (-128.86607, -73.23641) -> (-128.86607, -106.23641) construction
  line L12 (-137.86607, -106.23641) -> (-137.86607, -73.23641) construction
  line L13 (-137.86607, -73.23641) -> (-128.86607, -73.23641) construction
  line L14 (-119.66607, -106.23641) -> (-119.66607, -104.23641)
  line L15 (-119.66607, -104.23641) -> (-117.16607, -104.23641)
  line L16 (-117.16607, -104.23641) -> (-115.16607, -106.23641)
  line L17 (-119.66607, -104.23641) -> (-119.66607, -73.23641)
  line L18 (-119.66607, -73.23641) -> (-128.86607, -73.23641)
  line L19 (-140.56607, -104.23641) -> (-142.56607, -106.23641)
  line L20 (-138.06607, -104.23641) -> (-140.56607, -104.23641)
  line L21 (-138.06607, -104.23641) -> (-138.06607, -73.23641)
  line L22 (-138.06607, -106.23641) -> (-138.06607, -104.23641)
  line L23 (-138.06607, -73.23641) -> (-128.86607, -73.23641)
  line L24 (-119.86607, -69.87641) -> (-137.86607, -69.87641)
  line L25 (-119.66607, -104.73641) -> (-138.06607, -104.73641)
  line L26 (-119.86607, -69.87641) -> (-119.86607, -72.23641)
  line L27 (-119.86607, -72.23641) -> (-137.86607, -72.23641)
  line L28 (-137.86607, -72.23641) -> (-137.86607, -69.87641)
  point P0 (-128.86607, -106.23641)
  dimension "d82" = 33
  dimension "d83" = 18
  dimension "d84" = 45
  dimension "d85" = 2
  dimension "d86" = 2.5
  dimension "d87" = 0.2
  dimension "d93" = 1.5
  dimension "d102" = 1
  constraint perpendicular L5 L9
  constraint perpendicular L9 L10
  constraint perpendicular L5 L11
  constraint perpendicular L5 L14
  constraint perpendicular L14 L15
  constraint collinear L14 L17
  constraint tangent A2 L24
  constraint perpendicular L22 L25
  constraint perpendicular L24 L26
  constraint perpendicular L24 L28
  constraint perpendicular L27 L28
  constraint collinear L9 L26
  constraint collinear L12 L28
  measures "d83" distance of L9 L12
  measures "d84" angle of L8 L16
  measures "d93" distance of L5 L25
  measures "d102" distance of L18 L27
chamfer "Chamfer1" distance 1.8 angle 45 1 faces at (196.346904, 48.074498, 0) on bodies 1
chamfer "Chamfer1" distance 1.8 angle 45 1 faces at (153.499367, 59.091005, -1.4) on bodies 1
chamfer "Chamfer1" distance 0.4 angle 45 8 edges at (130.497643, 66.959237, 4) (130.497643, -20.670763, 4) (38.949075, -7.486293, 4) (19.590115, 86.727085, 4) (222.741583, -7.486293, 4) (305.407643, 36.629237, 4) (307.085832, 84.142675, 4) (243.778733, 84.810523, 4) on bodies 1
extrude "Extrude10" cut sketch "UCB-C cutout - fillet removal - profile" along normal up to surface (1.8 mm away) contours L5 L7 L8 L14 L22 L25 | L14 L17 L18 L21 L22 L23 L25 picked at (-127.169404, -105.23641) picked at (-128.86607, -93.903077) bodies 1
extrude "Extrude13" add sketch "UCB-C cutout - fillet removal - profile" along normal blind 1 from surface at 5.25 contours L5 L7 L8 L14 L22 L25 picked at (-127.169404, -105.23641) bodies 1
extrude "Extrude11" add sketch "UCB-C cutout - fillet removal - profile" along normal up to surface (6.25 mm away) contours L5 L8 L14 L15 L16 | L5 L8 L19 L20 L22 picked at (-117.332737, -105.569743) picked at (-140.399404, -105.569743) bodies 1
extrude "Extrude12" add sketch "UCB-C cutout - fillet removal - profile" along normal blind 3.5 draft 20 contours L24 L26 L27 L28 picked at (-128.86607, -71.449743) bodies 1
fillet "Fillet1" radius 1 4 edges at (133.95607, 107.23641, 5.25) (133.95607, 106.63641, 0.6) (123.77607, 107.23641, 5.25) (123.77607, 106.63641, 0.6) on bodies 1
sketch "Sketch13" plane through (0, 0, 0) normal (0, 0, 1) x (-1, 0, 0)
  line L0 (-138.06607, -104.23641) -> (-138.06607, -106.23641) construction
  line L1 (-138.06607, -106.23641) -> (-119.66607, -106.23641) construction
  line L2 (-119.66607, -106.23641) -> (-119.66607, -104.23641) construction
  line L3 (-103.957299, -29.011517) -> (-153.774841, -29.011517) construction
  line L4 (-153.774841, -29.011517) -> (-153.774841, -45.97641) construction
  line L5 (-153.774841, -45.97641) -> (-103.957299, -45.97641) construction
  line L6 (-103.957299, -45.97641) -> (-103.957299, -29.011517) construction
  line L7 (-128.86607, -66.32641) -> (-128.86607, 21.30359) construction
  line L8 (-137.86607, -69.87641) -> (-132.868569, -69.87641)
  arc A0 (-124.863571, -69.87641) -> (-132.868569, -69.87641) centre (-128.86607, -66.32641) ccw
  line L9 (-124.863571, -69.87641) -> (-119.86607, -69.87641)
  line L10 (-119.86607, -69.87641) -> (-119.86607, -72.23641)
  line L11 (-119.86607, -72.23641) -> (-137.86607, -72.23641)
  line L12 (-137.86607, -72.23641) -> (-137.86607, -69.87641)
  line L13 (-117.16607, -104.23641) -> (-116.96607, -104.43641)
  line L14 (-116.96607, -104.43641) -> (5.90393, -104.43641)
  arc A1 (5.90393, -104.43641) -> (8.10393, -102.23641) centre (5.90393, -102.23641) ccw
  line L15 (8.10393, -102.23641) -> (8.10393, 1.458095)
  arc A2 (8.10393, 1.458095) -> (6.472648, 3.583315) centre (5.90393, 1.458095) ccw
  line L16 (6.472648, 3.583315) -> (-112.893785, 35.52631)
  arc A3 (-112.893785, 35.52631) -> (-113.462504, 35.60109) centre (-113.462504, 33.40109) ccw
  line L17 (-113.462504, 35.60109) -> (-144.22489, 35.60109)
  arc A4 (-144.22489, 35.60109) -> (-144.789949, 35.527286) centre (-144.22489, 33.40109) ccw
  line L18 (-144.789949, 35.527286) -> (-269.657669, 2.342355)
  arc A5 (-272.174751, 2.01359) -> (-269.657669, 2.342355) centre (-272.174751, 11.81359) ccw
  line L19 (-272.174751, 2.01359) -> (-320.63607, 2.01359)
  arc A6 (-320.63607, 2.01359) -> (-322.83607, -0.18641) centre (-320.63607, -0.18641) ccw
  line L20 (-322.83607, -0.18641) -> (-322.83607, -102.23641)
  arc A7 (-322.83607, -102.23641) -> (-320.63607, -104.43641) centre (-320.63607, -102.23641) ccw
  line L21 (-320.63607, -104.43641) -> (-140.76607, -104.43641)
  line L22 (-140.76607, -104.43641) -> (-140.56607, -104.23641)
  line L23 (-140.56607, -104.23641) -> (-138.06607, -104.23641)
  line L24 (-119.66607, -104.23641) -> (-117.16607, -104.23641)
  circle A8 centre (-303.77607, -35.99641) radius 5.35
  circle A9 centre (-303.77607, -85.42641) radius 5.35
  circle A10 centre (-128.86607, 21.30359) radius 5.35
  circle A11 centre (-221.110011, 8.11912) radius 5.35
  circle A12 centre (-240.468971, -86.094258) radius 5.35
  circle A13 centre (-37.317502, 8.11912) radius 5.35
  circle A14 centre (-17.958543, -86.094258) radius 5.35
  point P0 (-128.86607, -45.97641)
  point P1 (-128.86607, -60.97641)
  dimension "d97" = 10
  dimension "d98" = 0
  dimension "d99" = 15
  text T0 "US8EK" font "Arial" height 10 align centre middle in box 49.817542 x 16.964893 at (-103.957299, -29.011517) x (-1, 0) y (0, -1) spacing 1 kerned
  constraint coincident L7